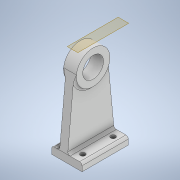
# Autodesk Inventor part: bracket
Saved by Autodesk Inventor 2021 (Build 250183000, 183)
## iProperties
Created: 2022-04-24
Part Number: bracket
Material: Generic
Document SubType Name: Modeling
Designer: hp
Density: 1 g/cm^3
Appearance: Default
Author: hp
Autodesk Inventor part; units mm, degrees
ref_plane "YZ Plane" through (0, 0, 0) normal (1, 0, 0) x (0, 1, 0)
ref_plane "XZ Plane" through (0, 0, 0) normal (0, 1, 0) x (-1, 0, 0)
ref_plane "XY Plane" through (0, 0, 0) normal (0, 0, 1) x (1, 0, 0)
sketch "Sketch1" plane through (0, 0, 0) normal (1, 0, 0) x (0, 1, 0)
  circle A0 centre (91.5, 0.099704) radius 13
  line L0 (9.5, 29) -> (0, 29)
  line L1 (0, 29) -> (0, -29)
  line L2 (0, -29) -> (9.5, -29)
  line L3 (9.5, -29) -> (9.5, 29)
  circle A1 centre (91.5, 0.099704) radius 21
  line L4 (9.5, 29) -> (93.489942, 21.005209)
  line L5 (93.539099, -20.801063) -> (9.5, -29)
  point P0 (0, 0)
  dimension "d0" = 58
  dimension "d1" = 29
  dimension "d2" = 9.5
  dimension "d3" = 26
  dimension "d4" = 42
  dimension "d5" = 82
  constraints: 12 end point, 2 centre point, 2 parallel, 2 point on circle, 2 tangent, 1 coincident, 1 horizontal, 1 perpendicular
  measures "d0" distance of L0.end L1.end
  measures "d1" distance from line of point (0, 0) L2
  measures "d2" distance from line of L3 point (0, 0)
  measures "d3" diameter of A0
  measures "d4" diameter of A1
  measures "d5" distance from line of L3 A0.centre
extrude "Extrusion1" add sketch "Sketch1" along normal blind 28 contours L3 L2 L1 L0
extrude "Extrusion2" add sketch "Sketch1" along normal blind 10 contours L4 A1 L5 L3
extrude "Extrusion3" add sketch "Sketch1" against normal blind 10 contours L3 L2 L1 L0
extrude "Extrusion4" add sketch "Sketch1" along normal blind 13 contours A1
extrude "Extrusion5" add sketch "Sketch1" against normal blind 3 contours A1
fillet "Fillet1" radius 3 1 edges at (10, 9.5, 0)
fillet "Fillet2" radius 3 1 edges at (0, 9.5, 0)
fillet "Fillet3" radius 3 1 edges at (0, 70.5, 0.075)
fillet "Fillet4" radius 3 1 edges at (10, 70.5, 0.075)
fillet "Fillet5" radius 3 1 edges at (28, 9.5, 0)
ref_plane "Work Plane1" through (13, 129.5, 29) normal (0, 1, 0) x (1, 0, 0)
sketch "Sketch2" plane through (13, 129.5, 29) normal (0, 1, 0) x (1, 0, 0)
  circle A0 centre (6, 48) radius 3
  line L0 (0, 58) -> (12, 58) projected
  line L1 (15, 0) -> (15, 58) projected
  circle A1 centre (6, 10) radius 3
  line L2 (0, 0) -> (12, 0) projected
  point P0 (-13, 29)
  dimension "d22" = 10
  dimension "d23" = 6
  dimension "d24" = 9
  dimension "d25" = 6
  dimension "d26" = 9
  dimension "d27" = 10
  constraints: 2 centre point
  measures "d22" distance from line of L0 A0.centre
  measures "d23" diameter of A0
  measures "d24" distance from line of L1 A0.centre
  measures "d25" diameter of A1
  measures "d26" distance from line of L1 A1.centre
  measures "d27" distance from line of L2 A1.centre
extrude "Extrusion6" cut sketch "Sketch2" against normal through all
fillet "Fillet6" radius 3 1 edges at (-10, 9.5, 0)
equation "\"d1\" = 0.5 * d0"
equation "\"d25\" = d23"
body "Solid1"
